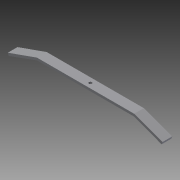
# Autodesk Inventor part: Frame
Saved by Autodesk Inventor 2015 (Build 190159000, 159)
## iProperties
Created: 2015-06-16
Part Number: Frame
Material: Generic
Document SubType Name: Modeling
Designer: david_000
Density: 1 g/cm^3
Appearance: Default
Author: david_000
Autodesk Inventor part; units mm, degrees
ref_plane "YZ Plane" through (0, 0, 0) normal (1, 0, 0) x (0, 1, 0)
ref_plane "XZ Plane" through (0, 0, 0) normal (0, 1, 0) x (-1, 0, 0)
ref_plane "XY Plane" through (0, 0, 0) normal (0, 0, 1) x (1, 0, 0)
sketch "Sketch1" plane through (0, 0, 0) normal (0, 0, 1) x (1, 0, 0)
  line L0 (0, 0) -> (127, 0)
  line L1 (127, 3.175) -> (0, 3.175)
  line L2 (0, 0) -> (-36.9784, -13.459)
  line L3 (0, 0) -> (39.3516, 0) construction
  line L4 (0, 3.175) -> (-38.1, -10.284)
  line L5 (-38.1, -10.284) -> (-36.9784, -13.459)
  line L6 (127, 3.175) -> (163.9784, -10.284)
  line L7 (127, 3.175) -> (166.3516, 3.175) construction
  line L8 (127, 0) -> (162.7842, -13.459)
  line L9 (162.7842, -13.459) -> (163.9784, -10.284)
  dimension "d0" = 127
  dimension "d1" = 3.175
  dimension "d2" = 160
  dimension "d3" = 20
  dimension "d4" = 38.1
  dimension "d5" = 127
  dimension "d6" = 3.175
  dimension "d7" = 3.175
  dimension "d8" = 0
  dimension "d9" = 0
  constraints: 20 end point, 3 horizontal, 2 equal length, 2 perpendicular, 1 parallel
  measures "d0" distance of L1.start L1.end
  measures "d1" distance of L0.end L1.start
  measures "d2" angle of L2 L3
  measures "d3" angle of L6 L7
  measures "d4" horizontal distance of L4.end L1.end
  measures "d5" distance of L0.start L0.end
  measures "d6" vertical distance of L8.end L6.end
  measures "d7" vertical distance of L4.end L2.end
  measures "d8" horizontal distance of L0.start L1.end
  measures "d9" vertical distance of L2.end L8.end
extrude "Extrusion1" add sketch "Sketch1" along normal blind 12.7
sketch "Sketch2" plane through (0, 3.175, 0) normal (0, 1, 0) x (1, 0, 0)
  line L0 (0, 0) -> (0, -12.7) projected
  line L1 (127, -12.7) -> (0, -12.7) projected
  point P0 (63.5, -6.35)
  dimension "d12" = 63.5
  dimension "d13" = 6.35
  measures "d12" distance from line of L0 point (63.5, -6.35)
  measures "d13" distance from line of L1 point (63.5, -6.35)
hole "Hole1" at (63.5, 3.175, 6.35) direction (0, -1, 0) diameter 3.683 end through all thread size "10-24 UNC" class "2B" standard "ANSI Unified Screw Threads"
body "Solid1"
